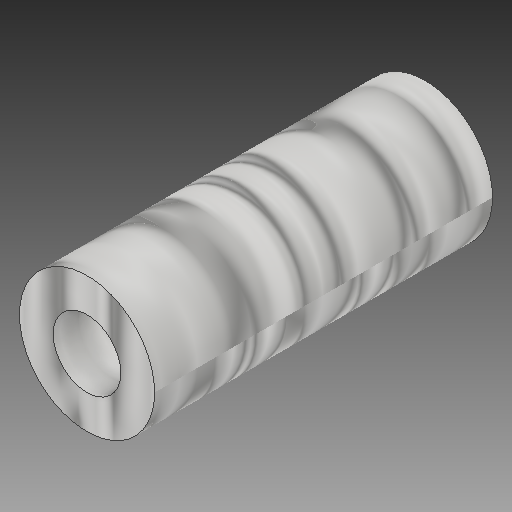
# Autodesk Inventor part: スペーサーm3,15
Saved by Autodesk Inventor 2020 (Build 240168000, 168)
## iProperties
Part Number: スペーサーm3,15
Material: アルミニウム 7075
Document SubType Name: Modeling
Designer: 雪村
Density: 2.81 g/cm^3
Appearance: サテン - ブラシ仕上げ 重厚
Mass: 0.893822 g
Surface Area: 4.66527 cm^2
Volume: 0.318086 cm^3
Author: 雪村
Autodesk Inventor part; units mm, degrees
ref_plane "YZ Plane" through (0, 0, 0) normal (1, 0, 0) x (0, 1, 0)
ref_plane "XZ Plane" through (0, 0, 0) normal (0, 1, 0) x (-1, 0, 0)
ref_plane "XY Plane" through (0, 0, 0) normal (0, 0, 1) x (1, 0, 0)
sketch "スケッチ1" plane through (0, 0, 0) normal (0, 0, 1) x (1, 0, 0)
  circle A0 centre (0, 0) radius 1.5
  circle A1 centre (0, 0) radius 3
  dimension "d0" = 3
  dimension "d1" = 6
  constraints: 2 centre point, 2 coincident
  measures "d0" diameter of A0
  measures "d1" diameter of A1
extrude "押し出し1" add sketch "スケッチ1" along normal blind 15
